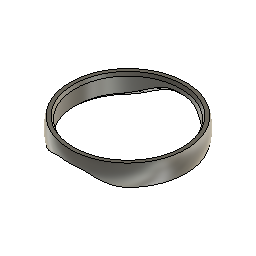
model (Autodesk Fusion 360 design; units mm, degrees)
Autodesk Fusion 360 part; units mm, degrees
sketch "Sketch1" plane through (0, 0, 0) normal (0, 1, 0) x (1, 0, 0)
  line L0 (0, 0) -> (0, -3) construction
  line L1 (0, -3) -> (-1, -3) construction
  line L2 (-1, -3) -> (-1, 0) construction
  line L3 (-1, 0) -> (0, 0) construction
  line L4 (0, 0) -> (7.5, 0) construction
  line L5 (0, -2.6) -> (-0.25, -3)
  line L6 (-0.75, -3) -> (-0.25, -3)
  line L7 (-1, -1.5) -> (0, -1.5) construction
  arc A0 (-1, -1.5) -> (-0.75, -3) centre (3.625, -1.5) ccw
  line L8 (0, -2.6) -> (0, -1.5)
  arc A1 (-0.75, 0) -> (-1, -1.5) centre (3.625, -1.5) ccw
  line L9 (-0.75, 0) -> (-0.25, 0)
  line L10 (0, -0.4) -> (-0.25, 0)
  line L11 (0, -0.4) -> (0, -1.5)
  line L12 (7.5, 0) -> (7.5, -1.5) construction
  line L13 (0, -2.6) -> (0, -3)
  line L14 (-0.25, -3) -> (0, -3)
  line L15 (0, 0) -> (0, -0.4)
  line L16 (0, 0) -> (-0.25, 0)
  dimension "d1" = 3
  dimension "d2" = 1
  dimension "d3" = 7.5
  dimension "d4" = 0.25
  dimension "d5" = 0.25
  dimension "d6" = 0.4
  constraint coincident L0.start L3.end
  constraint vertical L2
  constraint horizontal L1
  constraint vertical L0
  constraint horizontal L3
  constraint perpendicular L0 L4
  constraint coincident L0 L5.start
  constraint coincident L1 L5.end
  constraint coincident L1 L6.start
  constraint midpoint L2 L7.start
  constraint midpoint L0 L7.end
  constraint tangent L2 A0
  constraint symmetric L5.start L7 L10.start
  constraint symmetric L5.end L7 L9.end
  constraint symmetric L6.start L7 A1.start
  constraint symmetric A0.start L7 A1.end
  constraint symmetric L8.end L7 L11.end
  constraint symmetric L7 A0 A1
  constraint vertical L12
  constraint coincident L7 L12.end
  measures "d1" distance of L1.end L2.end
  measures "d2" distance of L0.end L1.end
  measures "d3" distance of L0.start L4.end
  measures "d4" distance of L0.end L5.end
  measures "d5" distance of L1.end L6.start
  measures "d6" distance of L0.end L5.start
revolve "Revolve1" add sketch "Sketch1" angle 360 about axis through (7.5, 0, 0) along (0, 0, 1) contours L5 L6 A0 L8 A1 L9 L10 L11 | L10 L15 L16
sketch "Sketch2" plane through (0, 0, 0) normal (0, 1, 0) x (1, 0, 0)
  line L0 (15.75, -3) -> (-0.75, -3)
  line L1 (15.75, 0) -> (-0.75, 0)
  arc A0 (4.8178, -1.1291) -> (6.5, -1.5) centre (6.5, 2.5) ccw
  line L2 (6.5, -1.5) -> (7.5, -1.5)
  line L3 (0, 0) -> (7.5, 0)
  line L4 (4.8178, -1.1291) -> (3.1822, -0.3709)
  arc A1 (3.1822, -0.3709) -> (1.5, 0) centre (1.5, -4) ccw
  line L5 (7.5, 0) -> (7.5, -1.5)
  line L6 (8.5, -1.5) -> (7.5, -1.5)
  arc A2 (8.5, -1.5) -> (10.1822, -1.1291) centre (8.5, 2.5) ccw
  line L7 (10.1822, -1.1291) -> (11.8178, -0.3709)
  arc A3 (13.5, 0) -> (11.8178, -0.3709) centre (13.5, -4) ccw
  point P0 (7.5, -1.5)
  dimension "d10" = 1
  dimension "d11" = 4
  dimension "d12" = 4
  dimension "d13" = 6
  constraint horizontal L2
  constraint tangent A0 L2
  constraint coincident P0 L2.end
  constraint tangent A0 L4
  constraint coincident L1 A1.end
  constraint tangent L4 A1
  constraint tangent L3 A1
  constraint symmetric A0.start L5 A2.end
  constraint symmetric A0.end L5 L6.start
  constraint symmetric A0 L5 A2
  constraint symmetric P0 L5 L2.end
  constraint symmetric L4.end L5 L7.end
  constraint symmetric A1.end L5 A3.start
  constraint symmetric A1 L5 A3
  measures "d10" distance of A0.end P0
  measures "d11" radius of A0
  measures "d12" radius of A1
  measures "d13" horizontal distance of P0 A1.end
extrude "Extrude1" cut sketch "Sketch2" against normal blind 11.5
pattern_circular "C-Pattern1" count 2 over 360 about axis through (7.5, 0, 0) along (0, 0, 1) of "Extrude1"
chamfer "Chamfer1" distance 0.5 angle 45 10 edges at (5.6408, 7.265, 1.4056) (3.973, 6.6189, 0.7375) (11.027, 6.6189, 0.7375) (9.3592, 7.265, 1.4056) (7.5, 7.5, 1.5) (9.3592, -7.265, 1.4056) (11.027, -6.6189, 0.7375) (3.973, -6.6189, 0.7375) (5.6408, -7.265, 1.4056) (7.5, -7.5, 1.5)
equation "d5 = d4"
